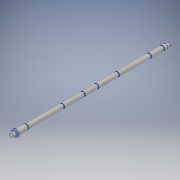
# Autodesk Inventor part: Column Axle
Saved by Autodesk Inventor 2019.4 (Build 234330000, 330)
## iProperties
Created: 2020-01-23
Part Number: Column Axle
Material: Aluminum 6061
Document SubType Name: Modeling
Designer: admin
Density: 2.7 g/cm^3
Appearance: Aluminum - Flat
Author: admin
Autodesk Inventor part; units mm, degrees
ref_plane "YZ Plane" through (0, 0, 0) normal (1, 0, 0) x (0, 1, 0)
ref_plane "XZ Plane" through (0, 0, 0) normal (0, 1, 0) x (-1, 0, 0)
ref_plane "XY Plane" through (0, 0, 0) normal (0, 0, 1) x (1, 0, 0)
sketch "Sketch1" plane through (0, 0, 0) normal (1, 0, 0) x (0, 1, 0)
  line L0 (0, 0) -> (2.5, 0)
  line L1 (2.5, 0) -> (2.5, -4)
  line L2 (2.5, -4) -> (3.5, -4)
  line L3 (3.5, -4) -> (3.5, -4.9)
  line L4 (3.5, -4.9) -> (4.6, -4.9)
  line L5 (4.6, -4.9) -> (4.6, -6)
  line L6 (4.6, -6) -> (3.5, -6)
  line L7 (3.5, -6) -> (3.5, -18.649)
  line L8 (3.5, -18.649) -> (2.65, -18.649)
  line L9 (3, -65.9) -> (2.65, -65.9)
  line L10 (2.65, -65.9) -> (2.65, -67)
  line L11 (2.65, -67) -> (3, -67)
  line L12 (3, -67) -> (3, -93)
  line L13 (3, -93) -> (2.65, -93)
  line L14 (2.65, -93) -> (2.65, -94.1)
  line L15 (2.65, -94.1) -> (3, -94.1)
  line L16 (3, -94.1) -> (3, -110.8)
  line L17 (3, -110.8) -> (2.65, -110.8)
  line L18 (2.65, -110.8) -> (2.65, -111.9)
  line L19 (2.65, -111.9) -> (3, -111.9)
  line L20 (3, -111.9) -> (3, -137.9)
  line L21 (3, -137.9) -> (2.65, -137.9)
  line L22 (2.65, -137.9) -> (2.65, -139)
  line L23 (2.65, -139) -> (3, -139)
  line L24 (3, -139) -> (3, -179.9)
  line L25 (3, -179.9) -> (2.65, -179.9)
  line L26 (2.65, -179.9) -> (2.65, -181)
  line L27 (2.65, -181) -> (3, -181)
  line L28 (3, -181) -> (3, -197)
  line L29 (3, -197) -> (2.65, -197)
  line L30 (2.65, -197) -> (2.65, -198.1)
  line L31 (2.65, -198.1) -> (3, -198.1)
  line L32 (3, -198.1) -> (3, -202)
  line L33 (3, -202) -> (2.5, -202)
  line L34 (2.5, -202) -> (2.5, -206)
  line L35 (2.5, -206) -> (0, -206)
  line L36 (0, -206) -> (0, 0)
  line L37 (2.65, -18.649) -> (2.65, -19.749)
  line L38 (2.65, -19.749) -> (3, -19.749)
  line L39 (3, -19.749) -> (3, -65.9)
  dimension "d0" = 2.5
  dimension "d1" = 3.5
  dimension "d2" = 1.1
  dimension "d4" = 0.35
  dimension "d5" = 1.1
  dimension "d6" = 1.1
  dimension "d7" = 1.1
  dimension "d8" = 1.1
  dimension "d9" = 1.1
  dimension "d10" = 1.1
  dimension "d11" = 4
  dimension "d12" = 1.1
  dimension "d13" = 2
  dimension "d14" = 2.5
  dimension "d15" = 12.649
  dimension "d16" = 4
  dimension "d17" = 0.35
  dimension "d18" = 1.1
  dimension "d19" = 3
  dimension "d20" = 26
  dimension "d21" = 16
  dimension "d22" = 206
  dimension "d23" = 26
  dimension "d24" = 67
  dimension "d25" = 67
  dimension "d26" = 5
  constraints: 80 end point, 25 perpendicular, 22 point on line, 2 vertical, 1 collinear, 1 horizontal
  measures "d0" distance of L0.start L0.end
  measures "d1" distance between parallel lines of L36 L7
  measures "d2" distance of L5.end L6.end
  measures "d4" distance of L9.start L9.end
  measures "d5" distance of L9.end L10.end
  measures "d6" distance of L13.end L14.end
  measures "d7" distance of L17.end L18.end
  measures "d8" distance of L21.end L22.end
  measures "d9" distance of L25.end L26.end
  measures "d10" distance of L29.end L30.end
  measures "d11" distance of L0.end L1.end
  measures "d12" distance of L4.end L5.end
  measures "d13" distance between parallel lines of L2 L6
  measures "d14" distance between parallel lines of L36 L34
  measures "d15" distance of L6.end L7.end
  measures "d16" distance of L33.end L34.end
  measures "d17" distance of L37.end L38.end
  measures "d18" distance of L8.end L37.end
  measures "d19" distance between parallel lines of L36 L12
  measures "d20" distance of L11.end L12.end
  measures "d21" distance of L27.end L28.end
  measures "d22" distance of L35.end L0.start
  measures "d23" distance of L19.end L20.end
  measures "d24" distance between parallel lines of L0 L11
  measures "d25" distance from line of L35 L22.end
  measures "d26" distance between parallel lines of L33 L29
revolve "Revolution1" add sketch "Sketch1" angle 360 about axis through (0, 0, -206) along (0, 0, 1)
body "Solid1"
